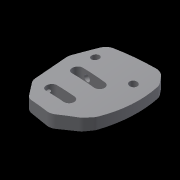
# Autodesk Inventor part: ThumbRouter
Saved by Autodesk Inventor 2015 (Build 190159000, 159)
## iProperties
Created: 2014-11-12
Part Number: ThumbRouter
Material: Generic
Document SubType Name: Modeling
Designer: Inventor
Density: 1 g/cm^3
Appearance: Default
Mass: 3.5521 g
Surface Area: 26.4028 cm^2
Volume: 3.5521 cm^3
RuleStatus: InUse
BeforeDocSave0: UpdateBoundingBox
CX: 29.98 mm
CY: 36.87 mm
CZ: 5.00 mm
Author: Inventor
Autodesk Inventor part; units mm, degrees
ref_plane "YZ Plane" through (0, 0, 0) normal (1, 0, 0) x (0, 1, 0)
ref_plane "XZ Plane" through (0, 0, 0) normal (0, 1, 0) x (-1, 0, 0)
sketch "Base" plane through (0, 0, 0) normal (0, 0, 1) x (1, 0, 0)
  circle A0 centre (-15.6718, 1.2221) radius 1.5
  circle A1 centre (-13.9696, -18.0615) radius 2
  line L0 (-13.9696, -18.0615) -> (-6.0134, -18.8977) construction
  circle A2 centre (-6.0134, -18.8977) radius 2
  circle A3 centre (-14.8088, -6.9127) radius 2
  circle A4 centre (-4.8636, -7.958) radius 2
  line L1 (-14.8088, -6.9127) -> (-4.8636, -7.958) construction
  line L2 (-14.1786, -20.0505) -> (-6.2224, -20.8868)
  line L3 (-13.7605, -16.0724) -> (-5.8043, -16.9087)
  line L4 (-15.0178, -8.9017) -> (-5.0726, -9.947)
  line L5 (-14.5997, -4.9237) -> (-4.6545, -5.9689)
  line L6 (-6.0134, -18.8977) -> (-4.8636, -7.958) construction
  circle A5 centre (1.2351, -0.5549) radius 1.5
  line L7 (-15.6718, 1.2221) -> (1.2351, -0.5549) construction
  line L8 (-21.3231, -18.1609) -> (-22.5392, -2.7087)
  line L9 (-15.0979, -25.987) -> (-21.3231, -18.1609)
  line L10 (-22.5392, -2.7087) -> (-17.4079, 7.5831)
  line L11 (-17.4079, 7.5831) -> (2.5, 9.5)
  line L12 (-4.7419, -27.72) -> (2.6752, -22.6223)
  line L13 (-15.0979, -25.987) -> (-4.7419, -27.72)
  arc A6 (4.998, -19.3658) -> (6.2351, 4.8044) centre (-36.6314, -5.1184) ccw
  line L14 (2.6752, -22.6223) -> (4.998, -19.3658)
  line L15 (2.5, 9.5) -> (6.2351, 4.8044)
  line L16 (-45.5436, 0) -> (16.8418, 0) construction
  line L17 (0, -35.164) -> (0, 16.944) construction
  dimension "d119" = 8
  dimension "d129" = 10
  dimension "d290" = 11
  dimension "d293" = 3
  dimension "d294" = 122
  dimension "d295" = 123
  dimension "d296" = 149
  dimension "d297" = 146
  dimension "d298" = 138
  dimension "d299" = 136
  dimension "d300" = 160
  dimension "d301" = 44
  dimension "d302" = 94.5
  dimension "d303" = 11.5
  dimension "d304" = 20
  dimension "d305" = 15.5
  dimension "d306" = 10
  dimension "d307" = 10.5
  dimension "d308" = 9
  dimension "d309" = 4
  dimension "d310" = 6
  dimension "d311" = 6
  dimension "d312" = 8
  dimension "d313" = 17
  dimension "d314" = 2.5
  dimension "d315" = 9.5
  dimension "d316" = 11
  dimension "d317" = 8
  dimension "d318" = 5
  dimension "d319" = 4
  constraints: 32 end point, 10 point on circle, 8 tangent, 7 centre point, 4 equal radius, 2 parallel, 1 coincident, 1 perpendicular
  measures "d119" distance of L0.start L0.end
  measures "d129" distance of L1.start L1.end
  measures "d290" distance between parallel lines of L0 L1
  measures "d293" diameter of A5
  measures "d294" angle of L11 L10
  measures "d295" angle of L11 L15
  measures "d296" angle of L8 L10
  measures "d297" angle of L9 L8
  measures "d298" angle of L13 L9
  measures "d299" angle of L12 L13
  measures "d300" angle of L14 L12
  measures "d301" radius of A6
  measures "d302" angle of L8 L16
  measures "d303" distance of L8.end L10.end
  measures "d304" distance of L10.end L11.end
  measures "d305" distance of L8.start L8.end
  measures "d306" distance of L9.start L8.start
  measures "d307" distance of L9.start L12.start
  measures "d308" distance of L12.start L12.end
  measures "d309" distance of L12.end L14.end
  measures "d310" distance of L11.end L15.end
  measures "d311" angle of L16 L1
  measures "d312" distance between parallel lines of L1 L7
  measures "d313" distance of L7.start L7.end
  measures "d314" distance from line of L11.end L17
  measures "d315" distance from line of L16 L11.end
  measures "d316" distance from line of L14.end L6
  measures "d317" distance from line of L9.start L0
  measures "d318" horizontal distance of L15.end L7.end
  measures "d319" diameter of A4
extrude "BaseFeature" add sketch "Base" along normal blind 5
fillet "BaseFilletsFeature" radius 4 9 edges at (6.2351, 4.8044, 2.5) (2.5, 9.5, 2.5) (4.998, -19.3658, 2.5) (2.6752, -22.6223, 2.5) (-4.7419, -27.72, 2.5) (-15.0979, -25.987, 2.5) (-21.3231, -18.1609, 2.5) (-22.5392, -2.7087, 2.5) (-17.4079, 7.5831, 2.5)
sketch "SideProfile" plane through (-15.2009, 7.7956, 5) normal (-0.0958, 0.9954, 0) x (0.9954, 0.0958, 0)
  arc A0 (-8.5605, 1.5) -> (21.6674, 1) centre (8.0701, 92.9423) ccw
  line L0 (21.6674, 1) -> (21.6674, 5)
  line L1 (21.6674, 5) -> (-8.5605, 5)
  line L2 (-8.5605, 1.5) -> (-8.5605, 5)
  line L3 (15.6109, 5) -> (0, 5) projected
  line L4 (15.6109, 0) -> (0, 0) construction
  line L5 (-8.5605, 0) -> (-8.5605, 5) projected
  line L6 (21.1674, 0) -> (21.1674, 5) projected
  dimension "d328" = 4
  dimension "d329" = 3.5
  dimension "d330" = 0.5
  constraints: 6 end point, 2 collinear, 2 point on circle, 2 vertical, 1 centre point, 1 perpendicular, 1 tangent
  measures "d328" distance of L0.start L0.end
  measures "d329" distance of L2.start L1.end
  measures "d330" distance between parallel lines of L0 L6
extrude "SideProfileFeature" cut sketch "SideProfile" against normal through all keep common part
sketch "ChannelAngle" plane through (0, 0, 0) normal (0, 0, -1) x (-1, 0, 0)
  line L0 (18.2542, -22.019) -> (7.4314, 8.5437) construction
  line L1 (20.5618, -19.1179) -> (16.0538, -24.7853) construction
  line L2 (-0.3382, 9.2918) -> (15.2009, 7.7956) construction
  line L3 (22.4522, -3.8145) -> (21.419, -16.9417) projected
  dimension "d331" = 156
  constraints: 2 end point, 1 midpoint, 1 point on line
  measures "d331" angle of L3 L0
ref_plane "ChannelAngleOrthoPlane" through (0.3382, 9.2918, 0) normal (-0.3338, -0.9426, 0) x (0, 0, 1)
ref_plane "ChannelAngleBasePlane" through (-18.2542, -22.019, 0) normal (-0.9426, 0.3338, 0) x (0.3338, 0.9426, 0)
sketch "Channel" plane through (0.3382, 9.2918, 0) normal (-0.3338, -0.9426, 0) x (0, 0, 1)
  circle A0 centre (2, 7.4241) radius 1.25
  line L0 (0, 0) -> (0, 14.1483) construction
  line L1 (3.6483, 17.4241) -> (0, 17.4241) projected
  dimension "d334" = 2.5
  dimension "d335" = 2
  dimension "d336" = 10
  constraints: 1 centre point
  measures "d334" diameter of A0
  measures "d335" distance from line of L0 A0.centre
  measures "d336" distance from line of A0.centre L1
hole "ChannelHoleFeature" at (-6.6601, 11.7701, 2) direction (-0.3338, -0.9426, 0) diameter 2.5 end through all
